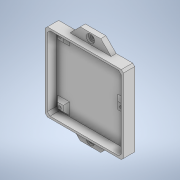
# Autodesk Inventor part: aluminium_block
Saved by Autodesk Inventor 2021 (Build 250183000, 183)
## iProperties
Created: 2020-07-08
Part Number: aluminium_block
Material: Generic
Document SubType Name: Modeling
Designer: OskarJohansson
Density: 1 g/cm^3
Appearance: Default
Author: OskarJohansson
## iProperties of the stored document _3DPrint.ipt
Created: 2020-08-06
Part Number: _3DPrint
Material: Generic
Document SubType Name: Modeling
Designer: OskarJohansson
Density: 1 g/cm^3
Appearance: Default
Author: OskarJohansson
Autodesk Inventor part; units mm, degrees
ref_plane "YZ Plane" through (0, 0, 0) normal (1, 0, 0) x (0, 1, 0)
ref_plane "XZ Plane" through (0, 0, 0) normal (0, 1, 0) x (-1, 0, 0)
ref_plane "XY Plane" through (0, 0, 0) normal (0, 0, 1) x (1, 0, 0)
sketch "Sketch1" plane through (0, 0, 0) normal (0, 0, 1) x (1, 0, 0)
  line L0 (-38, -38) -> (38, -38)
  line L1 (38, -38) -> (38, 38)
  line L2 (38, 38) -> (-38, 38)
  line L3 (-38, 38) -> (-38, -38)
  line L4 (-38, -38) -> (38, 38) construction
  line L5 (38, -38) -> (-38, 38) construction
  line L6 (-30, 35) -> (30, 35) projected
  line L7 (-35, -30) -> (-35, 30) projected
  line L8 (35, 30) -> (35, -30) projected
  line L9 (30, -35) -> (-30, -35) projected
  point P0 (0, 0)
  dimension "d0" = 3
  dimension "d1" = 3
  constraints: 12 end point, 2 midpoint, 2 parallel, 1 horizontal, 1 perpendicular
  measures "d0" distance between parallel lines of L2 L6
  measures "d1" distance between parallel lines of L1 L8
extrude "Extrusion1" add sketch "Sketch1" along normal blind 3 and the other way blind 5
sketch "Sketch2" plane through (0, 0, 3) normal (0, 0, 1) x (1, 0, 0)
  line L0 (35, -35) -> (-35, -35)
  line L1 (-35, -35) -> (-35, 35)
  line L2 (-35, 35) -> (35, 35)
  line L3 (35, 35) -> (35, -35)
  line L4 (35, -35) -> (-35, 35) construction
  line L5 (-35, -35) -> (35, 35) construction
  point P0 (0, 0)
  dimension "d6" = 70
  dimension "d7" = 70
  constraints: 12 end point, 2 midpoint, 2 parallel, 1 horizontal, 1 perpendicular
  measures "d6" distance of L0.end L1.end
  measures "d7" distance of L1.end L2.end
extrude "Extrusion2" cut sketch "Sketch2" against normal blind 6
sketch "Sketch3" plane through (0, 0, -3) normal (0, 0, 1) x (1, 0, 0)
  line L0 (-25, 25) -> (-35, 25)
  line L1 (-35, 25) -> (-35, 35)
  line L2 (-35, 35) -> (-25, 35)
  line L3 (-25, 35) -> (-25, 25)
  line L4 (-25, 25) -> (-35, 35) construction
  line L5 (-35, 25) -> (-25, 35) construction
  line L6 (-35, -35) -> (-35, 35) projected
  line L7 (-35, 35) -> (35, 35) projected
  point P0 (0, 0)
  point P1 (-30, 30)
  dimension "d10" = 10
  dimension "d11" = 10
  constraints: 12 end point, 2 collinear, 2 midpoint, 2 parallel, 1 horizontal, 1 perpendicular
  measures "d10" distance of L0.start L0.end
  measures "d11" distance of L2.end L0.start
extrude "Extrusion3" add sketch "Sketch3" along normal blind 3
sketch "Sketch4" plane through (0, 0, -3) normal (0, 0, 1) x (1, 0, 0)
  line L0 (25, -5) -> (35, -5)
  line L1 (35, -5) -> (35, 5)
  line L2 (35, 5) -> (25, 5)
  line L3 (25, 5) -> (25, -5)
  line L4 (25, -5) -> (35, 5) construction
  line L5 (35, -5) -> (25, 5) construction
  line L6 (-53.2, 0) -> (53.2, 0) projected
  line L7 (35, 35) -> (35, -35) projected
  point P0 (0, 0)
  point P1 (30, 0)
  point P2 (30, 0)
  dimension "d23" = 10
  dimension "d24" = 10
  constraints: 12 end point, 3 midpoint, 2 parallel, 1 collinear, 1 horizontal, 1 perpendicular, 1 point on line
  measures "d23" distance of L1.end L2.end
  measures "d24" distance of L0.end L1.end
extrude "Extrusion4" add sketch "Sketch4" along normal up to surface (3 mm away)
hole "Hole1" [suppressed]
mirror "Mirror1" about plane through (0, 0, 0) normal (0, 1, 0) of "Extrusion3"
chamfer "Chamfer1" distance 2 angle 45 8 edges at (38, 38, -1) (35, 35, 0) (38, -38, -1) (35, -35, 0) (-35, -35, 1.5) (-38, -38, -1) (-38, 38, -1) (-35, 35, 1.5)
thicken "Thicken1" operation add thickness 1 both sides no extend neighbours yes toward (0, 1, 0) faces at (13.6667, 35, 0) (-33.6667, 34.3333, 2) (-35, 8.3333, 2) (33.6667, 34.3333, 1) (35, -1.6667, 2) (33.6667, -34.3333, 1) (13.6667, -35, 0) (-34.3333, -33.6667, 2)
sketch "Sketch5" plane through (0, 0, -5) normal (0, 0, -1) x (-1, 0, 0)
  line L0 (10, -38) -> (-10, -38)
  line L1 (-10, -38) -> (-10, -48)
  line L2 (-10, -48) -> (10, -48)
  line L3 (10, -48) -> (10, -38)
  line L4 (10, -38) -> (-10, -48) construction
  line L5 (-10, -38) -> (10, -48) construction
  line L6 (36, -38) -> (-36, -38) projected
  line L7 (0, -65.2) -> (0, 55.2) construction
  line L8 (-10, -48) -> (-20, -38)
  line L9 (10, -48) -> (20, -38)
  point P0 (0, 0)
  point P1 (0, -43)
  point P2 (0, -43)
  dimension "d41" = 20
  dimension "d42" = 10
  dimension "d43" = 45
  constraints: 16 end point, 3 midpoint, 2 parallel, 2 point on line, 1 collinear, 1 horizontal, 1 perpendicular, 1 symmetric about line
  measures "d41" distance of L1.end L2.end
  measures "d42" distance of L0.end L1.end
  measures "d43" angle of L1 L8
extrude "Extrusion5" add sketch "Sketch5" against normal up to surface (5 mm away)
sketch "Sketch6" plane through (-10, -48, 0) normal (0, 0, 1) x (1, 0, 0)
  point P0 (10, 48)
  point P1 (10, 5)
hole "Hole4" at (0, -43, 0) direction (0, 0, -1) diameter 4.2 end through all counterbore diameter 8 counterbore depth 2
mirror "Mirror3" about plane through (0, 0, 0) normal (0, 1, 0) of "Extrusion5", "Hole4"
sketch "Sketch8" plane through (0, 0, 0) normal (0, 0, 1) x (1, 0, 0)
  line L0 (-53.2, 0) -> (53.2, 0) projected
  point P0 (0, 0)
  point P1 (30, 0)
  point P2 (-30, 30)
  point P3 (-30, -30)
  dimension "d64" = 60
  dimension "d65" = 30
  dimension "d66" = 30
  constraints: 1 point on line, 1 symmetric about line
  measures "d64" horizontal distance of point (-30, 30) point (30, 0)
  measures "d65" vertical distance of point (30, 0) point (-30, 30)
  measures "d66" distance of point (30, 0) point (0, 0)
hole "Hole5" at (30, 0, 0) at (-30, 30, 0) at (-30, -30, 0) direction (0, 0, -1) diameter 3 depth 3 tip angle 118
sketch "Sketch9" plane through (-36, -25, 0) normal (0, 0, 1) x (1, 0, 0)
  circle A0 centre (6, -5) radius 1.5 projected
  line L0 (0, -8.4142) -> (2.5858, -11) projected
  line L1 (11, -11) -> (2.5858, -11) projected
  line L2 (11, 0) -> (11, -11) projected
  line L3 (0, 0) -> (11, 0) projected
  line L4 (0, -8.4142) -> (0, 0) projected
  circle A1 centre (6, 55) radius 1.5 projected
  line L5 (2.5858, 61) -> (0, 58.4142) projected
  line L6 (0, 50) -> (0, 58.4142) projected
  line L7 (0, 50) -> (11, 50) projected
  line L8 (11, 50) -> (11, 61) projected
  line L9 (2.5858, 61) -> (11, 61) projected
  line L10 (11, 0) -> (2.5, 0)
  line L11 (2.5, 0) -> (2.5, -8.5)
  line L12 (2.5, -8.5) -> (11, -8.5)
  line L13 (11, -8.5) -> (11, 0)
  line L14 (11, 50) -> (0, 50) projected
  line L15 (11, 50) -> (2.5, 50)
  line L16 (2.5, 50) -> (2.5, 58.5)
  line L17 (2.5, 58.5) -> (11, 58.5)
  line L18 (11, 58.5) -> (11, 50)
  point P0 (36, 25)
  point P1 (11, -8.5)
  point P2 (2.5, 0)
  point P3 (11, 58.5)
  dimension "d74" = 3.5
  dimension "d75" = 3.5
  dimension "d81" = 3.5
  dimension "d82" = 3.5
  constraints: 16 end point, 4 parallel, 2 horizontal, 2 perpendicular
  measures "d74" distance from line of A0.centre L11
  measures "d75" distance from line of A0.centre L12
  measures "d81" distance from line of A1.centre L17
  measures "d82" distance from line of L16 A1.centre
extrude "Extrusion7" cut sketch "Sketch9" against normal up to surface (3 mm away) contours L4 L3 L11 L12 L2 L1 L0 | L9 L8 L17 L16 L7 L6 L5
chamfer "Chamfer2" distance 1.5 angle 45 22 edges at (-25, -29.25, -3) (-29.25, -25, -3) (-33.5, -29.25, -3) (-29.25, -33.5, -3) (-33.5, -29.25, 0) (-29.25, -25, 0) (-25, -29.25, 0) (-29.25, -33.5, 0) (-33.5, 29.25, 0) (-33.5, 29.25, -3) (-29.25, 25, 0) (-29.25, 25, -3) (-25, 29.25, 0) (-25, 29.25, -3) (-29.25, 33.5, 0) (-29.25, 33.5, -3) (30.5, -5, 0) (25, 0, -3) (25, 0, 0) (30.5, 5, 0) (30.5, 5, -3) (30.5, -5, -3)
move faces "Move1" translate (0, 0, 3) faces at (-11.1381, -37.3333, 3)
equation "\"d1\" = d0"
equation "\"d7\" = d6"
equation "\"d24\" = d23"
equation "\"d75\" = d74"
equation "\"d81\" = d74"
equation "\"d82\" = d74"
body "Solid1"
